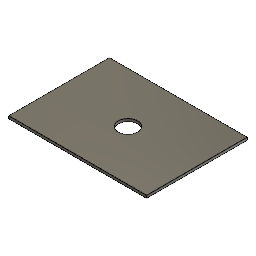
tapita (Autodesk Fusion 360 design; units mm, degrees)
Autodesk Fusion 360 part; units mm, degrees
sketch "Sketch1" plane through (0, 0, 0) normal (0, 1, 0) x (1, 0, 0)
  line L0 (0, 0) -> (50, 0)
  line L1 (50, 0) -> (50, 36.5)
  line L2 (50, 36.5) -> (0, 36.5)
  line L3 (0, 36.5) -> (0, 0)
  line L4 (0, 36.5) -> (50, 0)
  line L5 (50, 36.5) -> (0, 0)
  circle A0 centre (25, 18.25) radius 3.5
  dimension "d1" = 50
  dimension "d2" = 36.5
  dimension "d3" = 7
  measures "d2" distance of L0.start
  measures "d3" diameter of A0
extrude "Extrude1" add sketch "Sketch1" along normal blind 1 contours L0 L4 L5 A0 | L3 L4 L5 A0 | L1 L4 L5 A0 | L2 L4 L5 A0
